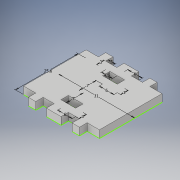
# Autodesk Inventor part: part_plunger_handle_side2
Saved by Autodesk Inventor 2017 (Build 210142000, 142)
## iProperties
Created: 2017-01-19
Part Number: part_plunger_handle_side2
Material: Generic
Document SubType Name: Modeling
Designer: John
Density: 1 g/cm^3
Appearance: Default
Author: John
Autodesk Inventor part; units mm, degrees
ref_plane "YZ Plane" through (0, 0, 0) normal (1, 0, 0) x (0, 1, 0)
ref_plane "XZ Plane" through (0, 0, 0) normal (0, 1, 0) x (-1, 0, 0)
ref_plane "XY Plane" through (0, 0, 0) normal (0, 0, 1) x (1, 0, 0)
sketch "Sketch2" plane through (0, 0, 0) normal (0, 1, 0) x (-1, 0, 0)
  line L0 (2.8786, -13.004) -> (2.8786, -16.004)
  line L1 (-3.1214, -13.004) -> (-3.1214, -16.004)
  line L2 (10.3786, -16.004) -> (10.3786, -13.004) construction
  line L3 (7.3786, -13.004) -> (7.3786, -16.004)
  line L4 (-7.6214, -16.004) -> (-7.6214, -13.004)
  line L5 (-10.6214, -13.004) -> (-10.6214, -16.004)
  line L6 (15.3786, -13.004) -> (15.3786, 12.596)
  line L7 (10.3786, 15.596) -> (10.3786, 12.5963)
  line L8 (7.3786, 12.596) -> (7.3786, 15.596)
  line L9 (2.8786, 15.7558) -> (2.8786, 12.596)
  line L10 (-3.1214, 12.7558) -> (-3.1214, 15.7558)
  line L11 (-7.6214, 15.7558) -> (-7.6214, 12.7558)
  line L12 (-10.6214, 12.596) -> (-10.6214, 15.7558)
  line L13 (10.3786, -16.004) -> (10.3786, -13.004)
  line L14 (15.3786, -13.004) -> (10.3786, -13.004)
  line L15 (10.3786, -16.004) -> (7.3786, -16.004)
  line L16 (7.3786, -13.004) -> (2.8786, -13.004)
  line L17 (2.8786, -16.004) -> (-3.1214, -16.004)
  line L18 (-3.1214, -13.004) -> (-7.6214, -13.004)
  line L19 (-7.6214, -16.004) -> (-10.6214, -16.004)
  line L20 (-10.6214, -13.004) -> (-15.6214, -13.004)
  line L21 (-15.6214, 12.596) -> (-10.6214, 12.596)
  line L22 (-10.6214, 15.7558) -> (-7.6214, 15.7558)
  line L23 (-7.6214, 12.7558) -> (-3.1214, 12.7558)
  line L24 (-3.1214, 15.7558) -> (2.8786, 15.7558)
  line L25 (2.8786, 12.596) -> (7.3786, 12.596)
  line L26 (7.3786, 15.596) -> (10.3786, 15.596)
  line L27 (10.3786, 12.5963) -> (15.3786, 12.596)
  line L28 (-15.6214, 12.596) -> (-15.6214, -13.004)
  line L29 (15.3786, -0.204) -> (-15.6214, -0.204) construction
  line L30 (7.3786, -13.004) -> (7.3786, -0.204) construction
  line L31 (7.3786, -0.204) -> (7.3786, 12.596) construction
  line L32 (2.8786, -10.204) -> (-3.1214, -10.204)
  line L33 (-3.1214, -10.204) -> (-3.1214, -7.204)
  line L34 (-3.1214, -7.204) -> (2.8786, -7.204)
  line L35 (2.8786, -7.204) -> (2.8786, -10.204)
  line L36 (2.8786, 6.796) -> (-3.1214, 6.796)
  line L37 (-3.1214, 6.796) -> (-3.1214, 9.796)
  line L38 (-3.1214, 9.796) -> (2.8786, 9.796)
  line L39 (2.8786, 9.796) -> (2.8786, 6.796)
  dimension "d14" = 3
  dimension "d15" = 3
  dimension "d16" = 6
  dimension "d17" = 31
  dimension "d18" = 4.5
  dimension "d19" = 25.6
  dimension "d39" = 6
  dimension "d40" = 3
  dimension "d41" = 7
  dimension "d42" = 6
  dimension "d43" = 3
  dimension "d44" = 7
  constraints: 81 end point, 22 parallel, 18 equal length, 5 collinear, 4 perpendicular, 4 point on line, 3 horizontal, 2 midpoint, 1 coincident, 1 vertical, 2 other
  measures "d14" distance of L2.start L2.end
  measures "d15" distance of L2.start L3.end
  measures "d16" distance of L0.end L1.end
  measures "d17" distance between parallel lines of L28 L6
  measures "d18" distance of L3.start L0.start
  measures "d19" distance of L6.start L6.end
  measures "d39" distance of L33.end L34.end
  measures "d40" distance of L32.end L33.end
  measures "d41" distance between parallel lines of L29 L34
  measures "d42" distance of L37.end L38.end
  measures "d43" distance of L36.end L37.end
  measures "d44" distance between parallel lines of L29 L36
extrude "Extrusion1" add sketch "Sketch2" along normal blind 3 contours L0 L17 L1 L18 L4 L19 L5 L20 L28 L21 L12 L22 L11 L23 L10 L24 L9 L25 L8 L26 L7 L27 L6 L14 L13 L15 L3 L16 | L32 L33 L34 L35 | L36 L37 L38 L39
extrude "Extrusion2" cut sketch "Sketch2" along normal up to next contours L36 L37 L38 L39
extrude "Extrusion3" cut sketch "Sketch2" along normal up to next contours L32 L33 L34 L35
body "Solid1"
